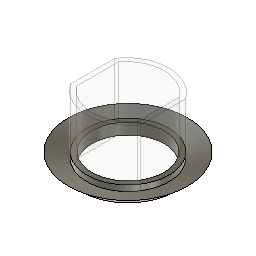
lock_shim (Autodesk Fusion 360 design; units mm, degrees)
Autodesk Fusion 360 part; units mm, degrees
sketch "Sketch1" plane through (0, 0, 0) normal (0, 0, 1) x (1, 0, 0) in component "Component"
  line L0 (0, 0) -> (0, 12)
  line L1 (19, 0) -> (19, 12)
  arc A0 (19, 12) -> (0, 12) centre (9.5, 5.5) ccw
  arc A1 (0, 0) -> (19, 0) centre (9.5, 6.5) ccw
  dimension "d1" = 12
  dimension "d2" = 12
  constraint coincident L0.start A1.start
  constraint vertical L0
  constraint vertical L1
  measures "d1" distance of L0.start L0.end
  measures "d2" distance of L1.end L1.start
extrude "Extrude1" add sketch "Sketch1" along normal blind 14 makes body 1 in component "Component"
sketch "Sketch2" plane through (0, 0, 14) normal (0, 0, 1) x (-1, 0, 0) in component "Component"
  arc A0 (0, 0) -> (-19, 0) centre (-9.5, -6.5) ccw
  line L0 (-19, 0) -> (-19, -12)
  arc A1 (-19, -12) -> (0, -12) centre (-9.5, -5.5) ccw
  line L1 (0, -12) -> (0, 0)
  line L2 (-1.3, -11.5846) -> (-1.3, -0.4155)
  arc A2 (-1.3, -0.4155) -> (-17.7, -0.4155) centre (-9.5, -6.5) ccw
  line L3 (-17.7, -0.4155) -> (-17.7, -11.5846)
  arc A3 (-17.7, -11.5846) -> (-1.3, -11.5846) centre (-9.5, -5.5) ccw
  dimension "d5" = -1.3
extrude "Extrude2" cut sketch "Sketch2" against normal blind 14 contours L2 A2 L3 A3 bodies 1 in component "Component"
sketch "Sketch1 (2)" plane through (0, 0, 0) normal (0, 0, 1) x (1, 0, 0) in component "Component'"
sketch "Sketch2 (2)" plane through (0, 0, 0) normal (1, 0, 0) x (0, 1, 0) in component "Component'"
  line L0 (-9.7, 0) -> (-9.7, -3)
  line L1 (-16, -0.1) -> (-12.661, -3)
  line L2 (-12.661, -3) -> (-9.7, -3)
  line L3 (-11, 0) -> (-11, -1.55)
  line L4 (-11, -1.55) -> (-16, -0.1)
  line L5 (-11, 0) -> (-9.7, 0)
  constraint vertical L0
  constraint perpendicular L0 L2
  constraint perpendicular L2 L3
  constraint perpendicular L0 L5
revolve "Revolve1" add sketch "Sketch2 (2)" angle 360 about axis through (0, 0, 1.75) along (0, 0, 1) separate body makes body 2 in component "Component'"
extrude "Extrude3" add 1 faces at (0.4333, 4.1385, 0) along direction (0, 0, -1) blind 3 on bodies 1 bodies 1 in component "Component"
component "Component" placed x (1, 0, 0) y (0, 1, 0) z (0, 0, 1) at (0, 0, 0)
component "Component'" placed x (1, 0, 0) y (0, 1, 0) z (0, 0, 1) at (9.5, 6, 0)
